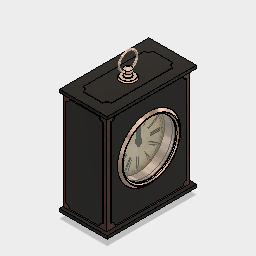
WoodenClock (Autodesk Fusion 360 design; units mm, degrees)
Autodesk Fusion 360 part; units mm, degrees
sketch "Base" plane through (0, 0, 0) normal (0, 1, 0) x (1, 0, 0)
  line L0 (-40, 75) -> (40, 75)
  line L1 (40, 75) -> (40, -75)
  line L2 (40, -75) -> (-40, -75)
  line L3 (-40, -75) -> (-40, 75)
  line L4 (20.4023, 0) -> (59.5977, 0) construction
  line L5 (0, -75) -> (0, 75) construction
  dimension "d1" = 80
  dimension "d2" = 150
  measures "d1" distance of L0.start L0.end
  measures "d2" distance of L0.start L2.end
extrude "Extrude1" add sketch "Base" along normal blind 5 makes body 1
sketch "Sketch2" plane through (0, 5, 0) normal (0, 1, 0) x (-1, 0, 0)
  line L0 (40, 75) -> (-40, 75)
  line L1 (-40, 75) -> (-40, -75)
  line L2 (-40, -75) -> (40, -75)
  line L3 (40, -75) -> (40, 75)
  line L4 (38, -70) -> (-34, -70)
  line L5 (-34, -70) -> (-34, 70)
  line L6 (-34, 70) -> (38, 70)
  line L7 (38, 70) -> (38, -70)
  dimension "d5" = 72
  dimension "d6" = 140
  dimension "d7" = 5
  dimension "d8" = 6
  measures "d5" distance of L4.start L4.end
  measures "d6" distance of L4.start L6.end
  measures "d7" distance of L0 L6
  measures "d8" distance of L1 L5
extrude "Extrude2" add sketch "Sketch2" along normal blind 168 separate body contours L4 L5 L6 L7 makes body 2
sketch "Sketch3" plane through (0, 173, 0) normal (0, 1, 0) x (-1, 0, 0)
  line L0 (38, 70) -> (-34, 70)
  line L1 (-34, 70) -> (-34, -70)
  line L2 (-34, -70) -> (38, -70)
  line L3 (38, -70) -> (38, 70)
  line L4 (40, -75) -> (-40, -75)
  line L5 (-40, -75) -> (-40, 75)
  line L6 (-40, 75) -> (40, 75)
  line L7 (40, 75) -> (40, -75)
  point P0 (40, -75)
  point P1 (-40, 75)
extrude "Extrude3" add sketch "Sketch3" along normal blind 5 separate body contours L0 L1 L2 L3 | L4 L5 L6 L7 makes body 3
sketch "Sketch4" plane through (0, 178, 0) normal (0, 1, 0) x (-1, 0, 0)
  line L0 (40, 75) -> (-40, 75)
  line L1 (-40, 75) -> (-40, -75)
  line L2 (-40, -75) -> (40, -75)
  line L3 (40, -75) -> (40, 75)
  circle A0 centre (0, 0) radius 13
  dimension "d13" = 26
  measures "d13" diameter of A0
extrude "Extrude4" add sketch "Sketch4" along normal blind 2 separate body contours A0 makes body 4
chamfer "Chamfer1" distance 2 angle 45 1 edges at (12.1203, 180, -4.701) on bodies 4
sketch "Sketch5" plane through (0, 0, 0) normal (0, 0, 1) x (1, 0, 0)
  line L0 (13, 178) -> (-13, 178)
  line L1 (0, 161) -> (0, 199) construction
  line L2 (-20, 194) -> (28, 194) construction
  line L3 (-11, 180) -> (11, 180)
  line L4 (0, 194) -> (-1.5, 194)
  line L5 (-27, 191) -> (48, 191) construction
  line L6 (-6, 199) -> (-6, 186) construction
  line L7 (-27, 186) -> (48, 186) construction
  line L8 (-27, 181) -> (48, 181) construction
  line L9 (-6, 188.9073) -> (-6, 165) construction
  line L10 (0, 180) -> (-6, 180)
  line L11 (-6, 180) -> (-6, 181)
  line L12 (-1.5, 194) -> (-6, 191)
  line L13 (-6, 191) -> (-6, 186)
  arc A0 (-6, 181) -> (-6, 186) centre (-6, 183.5) ccw
  line L14 (0, 194) -> (0, 180)
  dimension "d17" = 14
  dimension "d18" = 1.5
  dimension "d19" = 3
  dimension "d20" = 6
  dimension "d21" = 5
  dimension "d22" = 1
  measures "d17" distance of L2 L3
  measures "d18" distance of L4.start L4.end
  measures "d19" distance of L2 L5
  measures "d20" distance of L1 L6
  measures "d21" distance of L5 L7
  measures "d22" distance of L3 L8
revolve "Revolve1" add sketch "Sketch5" angle 360 about axis through (0, 161, 0) along (0, 1, 0) bodies 4
sketch "Sketch6" plane through (0, 0, 0) normal (0, 0, 1) x (1, 0, 0)
  circle A0 centre (0, 188.5) radius 1.75
  dimension "d24" = 3.5
  measures "d24" diameter of A0
extrude "Extrude5" cut sketch "Sketch6" along normal blind 8 and the other way blind 10 bodies 4
torus "TorusPrimitive1" add centre line diameter 30 section diameter 3 placed x (0, 0, -1) y (0, 1, 0) z (1, 0, 0) at (0, 205, 0) separate body makes body 5
move_body "MoveFace1" bodies 5 to x (1, 0, 0) y (0, 1, 0) z (0, 0, 1) at (0, -3, 0) on bodies 5
shell "Shell1" thickness 5 removed faces 2 at (-14, 173, -23.3333) at (-14, 5, -23.3333) on bodies 2
sketch "Sketch9" plane through (0, 0, 0) normal (0, -1, 0) x (1, 0, 0)
  line L0 (40, 75) -> (-40, 75)
  line L1 (-40, 75) -> (-40, -75)
  line L2 (-40, -75) -> (40, -75)
  line L3 (40, -75) -> (40, 75)
  line L4 (40, 75) -> (20, 75)
  line L5 (20, 75) -> (20, 55)
  line L6 (20, 55) -> (40, 55)
  line L7 (40, 55) -> (40, 75)
  line L8 (-40, 75) -> (-20, 75)
  line L9 (-20, 75) -> (-20, 55)
  line L10 (-20, 55) -> (-40, 55)
  line L11 (-40, 55) -> (-40, 75)
  line L12 (-40, -75) -> (-20, -75)
  line L13 (-20, -75) -> (-20, -55)
  line L14 (-20, -55) -> (-40, -55)
  line L15 (-40, -55) -> (-40, -75)
  line L16 (40, -75) -> (20, -75)
  line L17 (20, -75) -> (20, -55)
  line L18 (20, -55) -> (40, -55)
  line L19 (40, -55) -> (40, -75)
  dimension "d32" = 20
  dimension "d33" = 20
  dimension "d34" = 20
  dimension "d35" = 20
  dimension "d36" = 20
  dimension "d37" = 20
  dimension "d38" = 20
  dimension "d39" = 20
  measures "d32" distance of L0.start L6.end
  measures "d33" distance of L0.start L4.end
  measures "d34" distance of L0.end L8.end
  measures "d35" distance of L0.end L10.end
  measures "d36" distance of L1.end L12.end
  measures "d37" distance of L1.end L14.end
  measures "d38" distance of L2.end L18.end
  measures "d39" distance of L2.end L16.end
sphere "SpherePrimitive1" add diameter 20 placed x (1, 0, 0) y (0, 0, 1) z (0, -1, 0) at (-20, 0, 55) bodies 1
sphere "SpherePrimitive2" add diameter 20 placed x (1, 0, 0) y (0, 0, 1) z (0, -1, 0) at (20, 0, 55) bodies 1
sphere "SpherePrimitive3" add diameter 20 placed x (1, 0, 0) y (0, 0, 1) z (0, -1, 0) at (-20, 0, -55) bodies 1
sphere "SpherePrimitive4" add diameter 20 placed x (1, 0, 0) y (0, 0, 1) z (0, -1, 0) at (20, 0, -55) bodies 1
fillet "Fillet1" radius 2.5 4 edges at (16.3838, 0, 45.6767) (-23.6162, 0, 45.6767) (-23.6162, 0, -64.3233) (16.3838, 0, -64.3233) on bodies 1
sketch "Sketch10" plane through (34, 0, 0) normal (1, 0, 0) x (0, 0, -1)
  line L0 (-70, 5) -> (70, 5)
  line L1 (70, 5) -> (70, 173)
  line L2 (70, 173) -> (-70, 173)
  line L3 (-70, 173) -> (-70, 5)
  line L4 (-110.0929, 93) -> (140, 93) construction
  line L5 (75, 173) -> (-75, 173)
  line L6 (0, 240) -> (0, -23.5928) construction
  circle A0 centre (0, 93) radius 52.5
  circle A1 centre (0, 93) radius 45.5
  dimension "d45" = 80
  dimension "d46" = 105
  dimension "d53" = 7
  measures "d45" distance of L4 L5
  measures "d46" diameter of A0
  measures "d53" distance of A0 A1
extrude "Extrude7" add sketch "Sketch10" along normal blind 5 and the other way blind 20 separate body contours A0 | A1 makes body 6
extrude "Extrude8" cut sketch "Sketch10" along normal blind 10 and the other way blind 18 contours A1 bodies 2 6
chamfer "Chamfer2" distance 4 angle 45 1 edges at (39, 74.0152, 48.9472) on bodies 6
chamfer "Chamfer3" distance 2 angle 45 1 edges at (39, 109.4535, 42.4209) on bodies 6
extrude "Extrude9" add sketch "Sketch10" along normal blind 1 and the other way blind 1 separate body contours A1 makes body 7
move_face "OffsetFaces1" offset 0.15 1 faces at (30, 90.732, 45.4434) on bodies 6
sketch "Sketch11" plane through (34, 0, 0) normal (1, 0, 0) x (0, 0, -1)
  circle A0 centre (0, 93) radius 45.5
  line L0 (-70, 5) -> (70, 5)
  line L1 (70, 5) -> (70, 173)
  line L2 (70, 173) -> (-70, 173)
  line L3 (-70, 173) -> (-70, 5)
  line L4 (-63, 168) -> (63, 168)
  line L5 (63, 168) -> (63, 9)
  line L6 (63, 9) -> (-63, 9)
  line L7 (-63, 9) -> (-63, 168)
  line L8 (75, 173) -> (-75, 173)
  line L9 (-75, 5) -> (75, 5)
  circle A1 centre (-63, 168) radius 6
  circle A2 centre (63, 168) radius 6
  circle A3 centre (63, 9) radius 6
  circle A4 centre (-63, 9) radius 6
  circle A5 centre (0, 93) radius 53
  dimension "d67" = 5
  dimension "d68" = 4
  dimension "d69" = 7
  dimension "d70" = 7
  dimension "d71" = 12
  dimension "d72" = 12
  dimension "d73" = 12
  dimension "d74" = 12
  dimension "d75" = 106
  measures "d67" distance of L4 L8
  measures "d68" distance of L6 L9
  measures "d69" distance of L1 L5
  measures "d70" distance of L3 L7
  measures "d71" diameter of A1
  measures "d72" diameter of A2
  measures "d73" diameter of A3
  measures "d74" diameter of A4
  measures "d75" diameter of A5
extrude "Extrude11" add sketch "Sketch11" along normal blind 1.5 separate body contours L4 L5 L6 L7 A1 A2 A3 A4 makes body 8
sketch "Sketch12" plane through (0, 0, 70) normal (0, 0, 1) x (1, 0, 0)
  line L0 (-38, 5) -> (34, 5)
  line L1 (34, 5) -> (34, 173)
  line L2 (34, 173) -> (-38, 173)
  line L3 (-38, 173) -> (-38, 5)
  line L4 (-27, 168) -> (23, 168)
  line L5 (29, 162) -> (29, 15)
  line L6 (23, 9) -> (-27, 9)
  line L7 (-33, 15) -> (-33, 162)
  line L8 (-33, 5) -> (-33, 173)
  line L9 (-33, 5) -> (-33, 173)
  line L10 (29, 5) -> (29, 173)
  line L11 (40, 173) -> (-40, 173)
  line L12 (-40, 5) -> (40, 5)
  arc A0 (-33, 162) -> (-27, 168) centre (-33, 168) ccw
  arc A1 (23, 168) -> (29, 162) centre (29, 168) ccw
  arc A2 (29, 15) -> (23, 9) centre (29, 9) ccw
  arc A3 (33.4721, 5) -> (34, 5.6834) centre (29, 9) ccw
  arc A4 (-27, 9) -> (-33, 15) centre (-33, 9) ccw
  dimension "d78" = 5
  dimension "d79" = 4
  dimension "d81" = 5
  dimension "d83" = 5
  dimension "d85" = 12
  dimension "d87" = 12
  measures "d78" distance of L4 L11
  measures "d79" distance of L6 L12
  measures "d81" distance of L1 L5
  measures "d83" distance of L3 L7
  measures "d85" diameter of A1
  measures "d87" diameter of A2
extrude "Extrude12" add sketch "Sketch12" along normal blind 1.5 separate body contours L4 L5 L6 L7 L8 L9 L10 A0 A1 A2 A4 makes body 9
mirror "Mirror1" about plane through (0, 0, 0) normal (0, 0, 1) of bodies 9 makes body 10
sketch "Sketch13" plane through (0, 178, 0) normal (0, 1, 0) x (-1, 0, 0)
  line L0 (40, 75) -> (-40, 75)
  line L1 (-40, 75) -> (-40, -75)
  line L2 (-40, -75) -> (40, -75)
  line L3 (40, -75) -> (40, 75)
  line L4 (16.5, -59) -> (-16.5, -59)
  line L5 (-24, -51.5) -> (-24, 51.5)
  line L6 (-16.5, 59) -> (16.5, 59)
  line L7 (24, 51.5) -> (24, -51.5)
  arc A0 (24, -51.5) -> (16.5, -59) centre (24, -59) ccw
  arc A1 (-16.5, -59) -> (-24, -51.5) centre (-24, -59) ccw
  arc A2 (-24, 51.5) -> (-16.5, 59) centre (-24, 59) ccw
  arc A3 (16.5, 59) -> (24, 51.5) centre (24, 59) ccw
  dimension "d91" = 16
  dimension "d92" = 16
  dimension "d93" = 16
  dimension "d94" = 16
  dimension "d95" = 15
  dimension "d96" = 15
  dimension "d97" = 15
  dimension "d98" = 15
  measures "d91" distance of L2 L4
  measures "d92" distance of L0 L6
  measures "d93" distance of L3 L7
  measures "d94" distance of L1 L5
  measures "d95" diameter of A0
  measures "d96" diameter of A1
  measures "d97" diameter of A2
  measures "d98" diameter of A3
extrude "Extrude13" add sketch "Sketch13" along normal blind 0.3 draft -45 separate body contours L4 L5 L6 L7 A0 A1 A2 A3 makes body 11
combine "Combine1" operation add target body 3 tool bodies 11
fillet "Fillet2" radius 0.5 1 edges at (10.2556, 180, 3.9778) on bodies 4
fillet "Fillet3" radius 0.5 1 edges at (-5.594, 181, 2.1697) on bodies 4
fillet "Fillet4" radius 0.2 16 edges at (24, 178, 0) (18.6967, 178, 53.6967) (23.7, 178.3, 0) (18.4846, 178.3, 53.4846) (0, 178.3, 58.7) (0, 178, 59) (-18.6967, 178, 53.6967) (-18.4846, 178.3, 53.4846) (-23.7, 178.3, 0) (0, 178.3, -58.7) (18.4846, 178.3, -53.4846) (18.6967, 178, -53.6967) (-18.4846, 178.3, -53.4846) (-24, 178, 0) (-18.6967, 178, -53.6967) (0, 178, -59) on bodies 3
fillet "Fillet5" radius 0.1 12 edges at (-40, 178, 0) (0, 178, -75) (-40, 175.5, -75) (40, 178, 0) (40, 175.5, -75) (0, 173, -75) (0, 178, 75) (40, 173, 0) (40, 175.5, 75) (0, 173, 75) (-40, 175.5, 75) (-40, 173, 0) on bodies 3
fillet "Fillet6" radius 0.1 11 edges at (0, 5, 75) (-40, 5, 0) (0, 0, 75) (-40, 0, 0) (-40, 2.5, 75) (-40, 2.5, -75) (0, 5, -75) (0, 0, -75) (40, 2.5, -75) (40, 5, 0) (40, 0, 0) on bodies 1
fillet "Fillet7" radius 0.3 12 edges at (34, 5, 0) (-2, 5, -70) (34, 89, -70) (-38, 89, -70) (34, 89, 70) (-2, 5, 70) (-38, 89, 70) (-38, 5, 0) (-38, 173, 0) (-2, 173, 70) (34, 173, 0) (-2, 173, -70) on bodies 2
sphere "SpherePrimitive6" add diameter 1000 placed x (0, 0, -1) y (0, 1, 0) z (1, 0, 0) at (35, 93, 0) separate body makes body 12
move_body "MoveFace3" bodies 12 to x (1, 0, 0) y (0, 1, 0) z (0, 0, 1) at (-498, 0, 0) on bodies 12
ref_plane "WorkPlane2" through (34, 93, 0) normal (1, 0, 0) x (0, 0, -1)
split "Split2" by plane through (34, 93, 0) normal (1, 0, 0) bodies 12 makes body 13 at (36.4069, 105.6947, -20.774)
cylinder "CylinderPrimitive1" cut diameter 91 height 10 placed x (0, 0, -1) y (0, 1, 0) z (1, 0, 0) at (35, 93, 0) keep common part bodies 13
combine "Combine2" operation add target body 13 tool bodies 7
delete_body "RemoveBody1" bodies 12
cylinder "CylinderPrimitive2" cut diameter 4 height -15 placed x (0, 0, -1) y (0, 1, 0) z (1, 0, 0) at (16, 93, 0) bodies 6
cylinder "CylinderPrimitive3" add diameter 3.5 height -5 placed x (0, 0, -1) y (0, 1, 0) z (1, 0, 0) at (16, 93, 0) separate body makes body 14
move_face "OffsetFaces2" offset 4 1 faces at (16, 93.7935, 0.5833) on bodies 14
cylinder "CylinderPrimitive4" add diameter 6 height 0.5 placed x (0, 0, -1) y (0, 1, 0) z (1, 0, 0) at (20, 93, 0) bodies 14
sketch "Sketch21" plane through (16, 0, 0) normal (1, 0, 0) x (0, 0, -1)
  circle A0 centre (0, 93) radius 2
  circle A1 centre (0, 93) radius 45.35
ref_plane "WorkPlane3" through (18, 93, 0) normal (1, 0, 0) x (0, 0, -1)
sketch "HourArmSketch" plane through (18, 93, 0) normal (1, 0, 0) x (0, 0, -1)
  circle A0 centre (0, 0) radius 1.75
  circle A1 centre (0, 0) radius 1.75
  circle A2 centre (0, 0) radius 1.75
  circle A3 centre (0, 0) radius 1.75
  circle A4 centre (0, 0) radius 3.9002
  line L0 (1.0651, 8.8009) -> (3.6833, 1.2827)
  line L1 (3.6833, 1.2827) -> (1.0651, 8.8009)
  arc A5 (0.8886, 11.7871) -> (1.0651, 8.8009) centre (6.2474, 10.6056) ccw
  line L2 (0.7694, 10.2817) -> (0.8886, 11.7871)
  line L3 (1.9052, 16.3981) -> (0.8886, 11.7871)
  line L4 (1.5, 18.1) -> (1.9052, 16.3981)
  line L5 (1.9052, 16.3981) -> (1.5, 18.1)
  arc A6 (0.3, 19.5) -> (1.5, 18.1) centre (2.1478, 19.8696) ccw
  line L6 (0.3, 19.5) -> (0.2, 20)
  line L7 (0, 20) -> (0.2, 20)
  line L8 (0.2, 20) -> (0, 20)
  line L9 (2.0572, -3.3135) -> (1.3277, -3.7664)
  arc A7 (1.3277, -3.7664) -> (1.3277, -6.5) centre (2.1763, -5.1332) ccw
  line L10 (1.3277, -6.5) -> (1.3277, -7.0045)
  line L11 (1.3277, -6.5) -> (1.3277, -7.0045)
  arc A8 (0.8129, -6.7697) -> (0, -6.597) centre (0.0179, -8.5122) ccw
  line L12 (1.3277, -7.0045) -> (0.8129, -6.7697)
  line L13 (0, 0) -> (0, 28)
  line L14 (0, 23) -> (0.0179, -11.5978) construction
  arc A9 (0.0306, -6.5969) -> (-0.7821, -6.7705) centre (0.0147, -8.5122) ccw
  line L15 (-1.2967, -7.0059) -> (-0.7821, -6.7705)
  line L16 (-1.2972, -6.5014) -> (-1.2967, -7.0059)
  arc A10 (-1.2972, -6.5014) -> (-1.3, -3.7678) centre (-2.1472, -5.1355) ccw
  line L17 (-2.03, -3.3157) -> (-1.3, -3.7678)
  line L18 (-3.6608, 1.2789) -> (-1.0504, 8.7998)
  arc A11 (-1.0504, 8.7998) -> (-0.877, 11.7862) centre (-6.2345, 10.5991) ccw
  line L19 (-1.8984, 16.3962) -> (-0.877, 11.7862)
  line L20 (-1.8984, 16.3962) -> (-1.4949, 18.0984)
  arc A12 (-1.4949, 18.0984) -> (-0.2964, 19.4997) centre (-2.1446, 19.8673) ccw
  line L21 (-0.1969, 19.9998) -> (0.0031, 20)
  line L22 (-0.2964, 19.4997) -> (-0.1969, 19.9998)
  line L23 (0, 8) -> (1.5, 4.5)
  line L24 (1.5, 4.5) -> (0, 5)
  line L25 (1.5, 4.5) -> (0, 5)
  line L26 (-1.5, 4.5) -> (0, 8)
  line L27 (0, 18) -> (0.75, 16.25)
  line L28 (0, 18) -> (0.75, 16.25)
  line L29 (0.75, 16.25) -> (0, 14.5)
  line L30 (0.4907, 15.645) -> (0, 14.5)
  line L31 (-0.75, 16.25) -> (0, 18)
  line L32 (-0.75, 16.25) -> (0, 14.5)
  line L33 (-0.375, 15.375) -> (0, 14.5)
  line L34 (0, 5) -> (-1.5, 4.5)
  point P0 (3.6833, 1.2827)
  point P1 (0.8886, 11.7871)
  point P2 (1.9052, 16.3981)
  point P3 (1.5, 18.1)
  point P4 (0.2, 20)
  point P5 (0, 20)
  point P6 (2.0572, -3.3135)
  point P7 (1.3277, -3.7664)
  point P8 (1.3277, -7.0045)
  point P9 (0.8129, -6.7697)
  point P10 (0, 8)
  point P11 (1.5, 4.5)
  point P12 (0, 5)
  point P13 (-1.5, 4.5)
  point P14 (0, 18)
  point P15 (0.75, 16.25)
  point P16 (0, 14.5)
  point P17 (-0.75, 16.25)
extrude "Extrude14" add sketch "HourArmSketch" against normal blind 0.5 separate body contours A4 | A4 L0 L1 A5 L3 L4 L5 A6 L6 L7 L8 L13 L21 L23 L24 L25 L27 L28 L29 L30 | A4 L9 A7 L10 L11 A8 L12 A9 L15 L16 A10 L17 | A4 L13 L18 A11 L19 L20 A12 L21 L22 L26 L31 L32 L33 L34 | L13 L26 L34 | L13 L23 L24 L25 | L13 L31 L32 L33 | L13 L27 L28 L29 L30 makes body 15
extrude "Extrude15" cut sketch "HourArmSketch" against normal blind 1 contours L13 L26 L34 | L13 L23 L24 L25 | L13 L31 L32 L33 | L13 L27 L28 L29 L30 bodies 15
sketch "MinuteSketch" plane through (18, 93, 0) normal (1, 0, 0) x (0, 0, -1)
  circle A0 centre (0, 0) radius 3.9002
  line L0 (2.0572, -3.3135) -> (1.3277, -3.7664)
  arc A1 (1.3277, -3.7664) -> (1.3277, -6.5) centre (2.1763, -5.1332) ccw
  line L1 (1.3277, -6.5) -> (1.3277, -7.0045)
  line L2 (1.3277, -6.5) -> (1.3277, -7.0045)
  arc A2 (0.8129, -6.7697) -> (0, -6.597) centre (0.0179, -8.5122) ccw
  arc A3 (1.3277, -3.7664) -> (1.3277, -6.5) centre (2.1763, -5.1332) ccw
  circle A4 centre (0, 0) radius 1.75
  circle A5 centre (0, 0) radius 1.75
  circle A6 centre (0, 0) radius 1.75
  circle A7 centre (0, 0) radius 1.75
  circle A8 centre (0, 0) radius 3.9002
  arc A9 (1.3694, 25.364) -> (1.0941, 17.462) centre (22.2785, 20.6797) ccw
  line L3 (3.4783, 1.7644) -> (1.0941, 17.462)
  line L4 (1.3694, 25.364) -> (1.8639, 27.5714)
  line L5 (1.8639, 27.5714) -> (1.5, 29.1)
  arc A10 (0.7472, 30.2641) -> (1.5, 29.1) centre (2.595, 30.6336) ccw
  line L6 (0.7472, 30.2641) -> (0.2, 33)
  line L7 (0.2, 33) -> (0, 33)
  circle A11 centre (0, 0) radius 3.9002
  line L8 (0, 8) -> (1.5, 4.5)
  line L9 (0, 8) -> (1.5, 4.5)
  line L10 (-1.5, 4.5) -> (0, 5)
  line L11 (0, 5) -> (-1.5, 4.5)
  line L12 (0, 8) -> (-1.5, 4.5)
  line L13 (0, 5) -> (1.5, 4.5)
  line L14 (0, 18) -> (0.75, 16.25)
  line L15 (0.75, 16.25) -> (0, 14.5)
  line L16 (-0.75, 16.25) -> (0, 14.5)
  line L17 (0, 14.5) -> (-0.75, 16.25)
  line L18 (0, 18) -> (-0.75, 16.25)
  line L19 (0, 29.7158) -> (1, 27.5)
  line L20 (0, 29.7158) -> (1, 27.5)
  line L21 (0, 25.5) -> (1, 27.5)
  line L22 (-1, 27.5) -> (0, 25.5)
  line L23 (0, 29.7158) -> (-1, 27.5)
  line L24 (0, 37) -> (0, 12)
  line L25 (0, 36) -> (0, 22.5389) construction
  line L26 (-0.2, 33) -> (0, 33)
  line L27 (-0.7472, 30.2641) -> (-0.2, 33)
  arc A12 (-1.5, 29.1) -> (-0.7472, 30.2641) centre (-2.595, 30.6336) ccw
  line L28 (-1.8639, 27.5714) -> (-1.5, 29.1)
  line L29 (-1.3694, 25.364) -> (-1.8639, 27.5714)
  arc A13 (-1.0941, 17.462) -> (-1.3694, 25.364) centre (-22.2785, 20.6797) ccw
  line L30 (-3.4783, 1.7644) -> (-1.0941, 17.462)
  line L31 (-2.0572, -3.3135) -> (-1.3277, -3.7664)
  arc A14 (-1.3277, -6.5) -> (-1.3277, -3.7664) centre (-2.1763, -5.1332) ccw
  line L32 (-1.3277, -6.5) -> (-1.3277, -7.0045)
  arc A15 (0, -6.597) -> (-0.8129, -6.7697) centre (-0.0179, -8.5122) ccw
  line L33 (0.8129, -6.7697) -> (1.3277, -7.0045)
  line L34 (-0.8129, -6.7697) -> (-1.3277, -7.0045)
  point P0 (2.0572, -3.3135)
  point P1 (1.3277, -3.7664)
  point P2 (1.3277, -7.0045)
  point P3 (0.8129, -6.7697)
  point P4 (1.0941, 17.462)
  point P5 (1.8639, 27.5714)
  point P6 (1.5, 29.1)
  point P7 (0.2, 33)
  point P8 (0, 33)
  point P9 (0, 8)
  point P10 (1.5, 4.5)
  point P11 (0, 5)
  point P12 (-1.5, 4.5)
  point P13 (0, 18)
  point P14 (0.75, 16.25)
  point P15 (0, 14.5)
  point P16 (-0.75, 16.25)
  point P17 (0, 29.7158)
  point P18 (1, 27.5)
  point P19 (0, 25.5)
  point P20 (-1, 27.5)
extrude "Extrude16" add sketch "MinuteSketch" along normal blind -1.5 and the other way blind 1 separate body makes body 16
sketch "SecondsSketch" plane through (18, 93, 0) normal (1, 0, 0) x (0, 0, -1)
  line L0 (0, 43) -> (0.8853, 39.2067)
  arc A0 (0.4427, 36.9541) -> (0.8853, 39.2067) centre (-1.8358, 38.5717) ccw
  line L1 (0.4427, 36.9541) -> (1.3498, 14.2202)
  arc A1 (1.3498, 14.2202) -> (3, 3) centre (54.8317, 16.3544) ccw
  circle A2 centre (0, 0) radius 3.5273
  line L2 (3, 3) -> (3.4596, 0.6877)
  line L3 (2.2071, -2.7515) -> (0.9, -3.8)
  line L4 (0.9, -3.8) -> (0.7097, -3.9526)
  arc A3 (0.7097, -3.9526) -> (0.7097, -5.3) centre (1.2501, -4.6263) ccw
  line L5 (0.7097, -5.3) -> (0.8299, -5.3964)
  line L6 (0.7903, -5.4847) -> (0.3424, -5.4085)
  arc A4 (0.3424, -5.4085) -> (0, -5.5) centre (0.2711, -5.828) ccw
  arc A5 (0.7903, -5.4847) -> (0.8299, -5.3964) centre (0.7986, -5.4354) ccw
  line L7 (0, 16) -> (0, 4) construction
  arc A6 (0, -5.5) -> (-0.3424, -5.4085) centre (-0.2711, -5.828) ccw
  line L8 (-0.7903, -5.4847) -> (-0.3424, -5.4085)
  arc A7 (-0.8299, -5.3964) -> (-0.7903, -5.4847) centre (-0.7986, -5.4354) ccw
  line L9 (-0.7097, -5.3) -> (-0.8299, -5.3964)
  arc A8 (-0.7097, -5.3) -> (-0.7097, -3.9526) centre (-1.2501, -4.6263) ccw
  line L10 (-0.9, -3.8) -> (-0.7097, -3.9526)
  line L11 (-2.2071, -2.7515) -> (-0.9, -3.8)
  line L12 (-3, 3) -> (-3.4596, 0.6877)
  arc A9 (-3, 3) -> (-1.3498, 14.2202) centre (-54.8317, 16.3544) ccw
  line L13 (-0.4427, 36.9541) -> (-1.3498, 14.2202)
  line L14 (0, 43) -> (-0.8853, 39.2067)
  arc A10 (-0.8853, 39.2067) -> (-0.4427, 36.9541) centre (1.8358, 38.5717) ccw
  line L15 (0, 30) -> (1.0391, 3.9614)
  arc A11 (1.0391, 3.9614) -> (0, 4.0954) centre (0, 0) ccw
  line L16 (0, 30) -> (-1.0391, 3.9614)
  arc A12 (0, 4.0954) -> (-1.0391, 3.9614) centre (0, 0) ccw
  dimension "d127" = 0.05
  measures "d127" radius of A5
extrude "Extrude17" add sketch "SecondsSketch" along normal blind 1.5 and the other way blind -1 separate body contours L0 A0 L1 A1 A2 L2 L12 A9 L13 L14 A10 | A2 | A2 L3 L4 A3 L5 L6 A4 A5 A6 L8 A7 L9 A8 L10 L11 | L15 A11 L16 A12 makes body 17
extrude "Extrude18" cut sketch "SecondsSketch" along normal blind 9 contours L15 A11 L16 A12 bodies 17
sketch "Sketch29" plane through (19.5, 0, 0) normal (1, 0, 0) x (0, 0, -1)
  line L0 (0, 123) -> (1.0391, 96.9614)
  arc A0 (1.0391, 96.9614) -> (-1.0391, 96.9614) centre (0, 93) ccw
  line L1 (-1.0391, 96.9614) -> (0, 123)
  line L2 (0, 136) -> (-0.8853, 132.2067)
  arc A1 (-0.8853, 132.2067) -> (-0.4427, 129.9541) centre (1.8358, 131.5717) ccw
  line L3 (-0.4427, 129.9541) -> (-1.3498, 107.2202)
  arc A2 (-3, 96) -> (-1.3498, 107.2202) centre (-54.8317, 109.3544) ccw
  line L4 (-3, 96) -> (-3.4596, 93.6877)
  arc A3 (-3.4596, 93.6877) -> (-2.2071, 90.2485) centre (0, 93) ccw
  line L5 (-2.2071, 90.2485) -> (-0.7097, 89.0474)
  arc A4 (-0.7097, 87.7) -> (-0.7097, 89.0474) centre (-1.2501, 88.3737) ccw
  line L6 (-0.7097, 87.7) -> (-0.8299, 87.6036)
  arc A5 (-0.8299, 87.6036) -> (-0.7903, 87.5153) centre (-0.7986, 87.5646) ccw
  line L7 (-0.7903, 87.5153) -> (-0.3424, 87.5915)
  arc A6 (0, 87.5) -> (-0.3424, 87.5915) centre (-0.2711, 87.172) ccw
  arc A7 (0.3424, 87.5915) -> (0, 87.5) centre (0.2711, 87.172) ccw
  line L8 (0.3424, 87.5915) -> (0.7903, 87.5153)
  arc A8 (0.7903, 87.5153) -> (0.8299, 87.6036) centre (0.7986, 87.5646) ccw
  line L9 (0.8299, 87.6036) -> (0.7097, 87.7)
  arc A9 (0.7097, 89.0474) -> (0.7097, 87.7) centre (1.2501, 88.3737) ccw
  line L10 (0.7097, 89.0474) -> (2.2071, 90.2485)
  arc A10 (2.2071, 90.2485) -> (3.4596, 93.6877) centre (0, 93) ccw
  line L11 (3.4596, 93.6877) -> (3, 96)
  arc A11 (1.3498, 107.2202) -> (3, 96) centre (54.8317, 109.3544) ccw
  line L12 (1.3498, 107.2202) -> (0.4427, 129.9541)
  arc A12 (0.4427, 129.9541) -> (0.8853, 132.2067) centre (-1.8358, 131.5717) ccw
  line L13 (0.8853, 132.2067) -> (0, 136)
  circle A13 centre (0, 93) radius 1
  dimension "d134" = 2
  measures "d134" diameter of A13
extrude "Extrude19" cut sketch "Sketch29" along normal blind 15 and the other way blind 11 contours A13 bodies 17
ref_plane "WorkPlane1" through (34, 93, 0) normal (-1, 0, 0) x (0, 0, 1)
named bodies: "Bottom", "Body", "Holder", "Ring", "Top", "ClockFrame", "Glass", "FrontDeco", "LeftDeco", "RightDeco", "pin", "HourArm", "MinuteArm", "SecondsArm"
